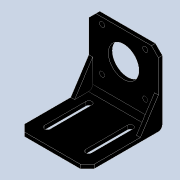
# Autodesk Inventor part: Nema 17 Stepper Motor Mounting Bracket
Saved by Autodesk Inventor 2022 (Build 260153000, 153)
## iProperties
Created: 2021-12-24
Part Number: Nema 17 Stepper Motor Mounting Bracket
Material: Generic
Document SubType Name: Modeling
Designer: Coy
Density: 1 g/cm^3
Appearance: Anodized - Black
Author: Coy
Autodesk Inventor part; units mm, degrees
ref_plane "YZ Plane" through (0, 0, 0) normal (1, 0, 0) x (0, 1, 0)
ref_plane "XZ Plane" through (0, 0, 0) normal (0, 1, 0) x (-1, 0, 0)
ref_plane "XY Plane" through (0, 0, 0) normal (0, 0, 1) x (1, 0, 0)
sketch "Sketch1" plane through (0, 0, 0) normal (1, 0, 0) x (0, 1, 0)
  line L0 (3, 0) -> (51, 0)
  line L1 (51, 0) -> (51, 2.85)
  line L2 (51, 2.85) -> (5.85, 2.85)
  line L3 (2.85, 5.85) -> (2.85, 54)
  line L4 (2.85, 54) -> (0, 54)
  line L5 (0, 54) -> (0, 3)
  arc A0 (0, 3) -> (3, 0) centre (3, 3) ccw
  arc A1 (2.85, 5.85) -> (5.85, 2.85) centre (5.85, 5.85) ccw
  point P0 (0, 0)
  dimension "d0" = 51
  dimension "d1" = 2.85
  dimension "d2" = 2.85
  dimension "d3" = 54
  dimension "d4" = 3
  constraints: 12 end point, 5 perpendicular, 4 point on circle, 4 tangent, 2 centre point, 2 point on line, 1 equal radius, 1 horizontal
  measures "d0" distance of point (0, 0) L0.end
  measures "d1" distance of L0.end L1.end
  measures "d2" distance of L3.end L4.end
  measures "d3" distance of L4.end point (0, 0)
  measures "d4" radius of A0
extrude "Extrusion1" add sketch "Sketch1" against normal blind 50
sketch "Sketch2" plane through (0, 0, 0) normal (1, 0, 0) x (0, 0, -1)
  line L0 (-54, 2.85) -> (-54, 0) projected
  line L1 (-54, 0) -> (-3, 0) projected
  arc A0 (-3, 0) -> (0, 3) centre (-3, 3) ccw projected
  line L2 (0, 3) -> (0, 51) projected
  line L3 (0, 51) -> (-2.85, 51) projected
  line L4 (-2.85, 51) -> (-2.85, 5.85) projected
  arc A1 (-5.85, 2.85) -> (-2.85, 5.85) centre (-5.85, 5.85) ccw projected
  line L5 (-5.85, 2.85) -> (-54, 2.85) projected
  line L6 (-5.85, 2.85) -> (-54, 2.85) projected
  line L7 (-15.85, 2.85) -> (-2.85, 22.85)
  line L8 (-2.85, 51) -> (-2.85, 5.85) projected
  point P0 (0, 0)
  point P1 (-2.85, 22.85)
  dimension "d7" = 20
  dimension "d8" = 13
  constraints: 2 end point, 2 point on line
  measures "d7" distance from line of L5 L7.end
  measures "d8" distance from line of L4 L7.start
extrude "Extrusion2" add sketch "Sketch2" against normal blind 2.8 contours L7 L4 A1 L5
sketch "Sketch3" plane through (-50, 0, 0) normal (-1, 0, 0) x (0, 0, 1)
  line L0 (2.85, 5.85) -> (2.85, 22.85) projected
  arc A0 (2.85, 5.85) -> (5.85, 2.85) centre (5.85, 5.85) ccw projected
  line L1 (15.85, 2.85) -> (5.85, 2.85) projected
  line L2 (15.85, 2.85) -> (2.85, 22.85) projected
  point P0 (0, 0)
extrude "Extrusion3" add sketch "Sketch3" against normal blind 2.8
sketch "Sketch4" plane through (0, 3, 0) normal (0, 0, -1) x (-1, 0, 0)
  line L0 (0, 48) -> (50, 48) construction
  line L1 (25, 48) -> (25, -3) construction
  line L2 (0, -3) -> (50, -3) construction
  line L3 (0, 48) -> (0, 19.85) construction
  line L4 (0, 28) -> (50, 28) construction
  line L5 (50, 48) -> (50, 0) construction
  circle A0 centre (25, 28) radius 11
  line L6 (9.5, 43.5) -> (40.5, 43.5) construction
  line L7 (40.5, 43.5) -> (40.5, 12.5) construction
  line L8 (40.5, 12.5) -> (9.5, 12.5) construction
  line L9 (9.5, 12.5) -> (9.5, 43.5) construction
  circle A1 centre (9.5, 43.5) radius 1.8
  circle A2 centre (40.5, 43.5) radius 1.8
  circle A3 centre (40.5, 12.5) radius 1.8
  circle A4 centre (9.5, 12.5) radius 1.8
  dimension "d13" = 20
  dimension "d14" = 22
  dimension "d15" = 31
  dimension "d16" = 31
  dimension "d17" = 3.6
  dimension "d18" = 3.6
  dimension "d19" = 3.6
  dimension "d20" = 3.6
  dimension "d21" = 15.5
  dimension "d22" = 15.5
  constraints: 12 end point, 5 centre point, 4 coincident, 3 midpoint, 2 horizontal, 2 parallel, 2 point on line, 1 perpendicular
  measures "d13" distance between parallel lines of L0 L4
  measures "d14" diameter of A0
  measures "d15" distance of L7.end L8.end
  measures "d16" distance of L6.end L7.end
  measures "d17" diameter of A1
  measures "d18" diameter of A2
  measures "d19" diameter of A3
  measures "d20" diameter of A4
  measures "d21" distance between parallel lines of L1 L7
  measures "d22" distance between parallel lines of L4 L6
extrude "Extrusion4" cut sketch "Sketch4" against normal up to next
sketch "Sketch5" plane through (0, 0, 3) normal (0, -1, 0) x (1, 0, 0)
  line L0 (0, 51) -> (-50, 51) construction
  line L1 (-38.7, -3) -> (-42.3, -3) construction
  line L2 (-39.85, 51) -> (-39.85, -3.09) construction
  line L3 (0, -3) -> (-50, -3) construction
  line L4 (-50, 0) -> (-50, 51) construction
  line L5 (-25, 51) -> (-25, -3) construction
  line L6 (-39.85, 42) -> (-39.85, 7.75) construction
  line L7 (-42, 39.85) -> (-42, 9.9)
  line L8 (-37.7, 9.9) -> (-37.7, 39.85)
  arc A0 (-37.7, 39.85) -> (-42, 39.85) centre (-39.85, 39.85) ccw
  arc A1 (-42, 9.9) -> (-37.7, 9.9) centre (-39.85, 9.9) ccw
  line L9 (-10.15, 42) -> (-10.15, 7.75) construction
  line L10 (-8, 39.85) -> (-8, 9.9)
  line L11 (-12.3, 9.9) -> (-12.3, 39.85)
  arc A2 (-8, 39.85) -> (-12.3, 39.85) centre (-10.15, 39.85) ccw
  arc A3 (-12.3, 9.9) -> (-8, 9.9) centre (-10.15, 9.9) ccw
  point P0 (-39.85, 24.875)
  point P1 (-10.15, 24.875)
  dimension "d25" = 10.15
  dimension "d26" = 34.25
  dimension "d27" = 4.3
  dimension "d28" = 9
  constraints: 20 end point, 12 point on circle, 9 symmetric about line, 7 point on line, 4 centre point, 4 tangent, 3 midpoint, 1 parallel, 1 perpendicular, 2 other
  measures "d25" distance between parallel lines of L4 L2
  measures "d26" distance of L6.start L6.end
  measures "d27" diameter of A1
  measures "d28" distance from line of L0 L6.start
extrude "Extrusion5" cut sketch "Sketch5" against normal up to next
chamfer "Chamfer1" distance 5 angle 45 4 edges at (0, 1.425, 54) (-50, 1.425, 54) (-50, 51, 1.425) (0, 51, 1.425)
equation "\"d2\" = d1"
equation "\"d18\" = d17"
equation "\"d19\" = d17"
equation "\"d20\" = d17"
equation "\"d21\" = 0.5 * d15"
equation "\"d22\" = 0.5 * d16"
body "Solid1"
